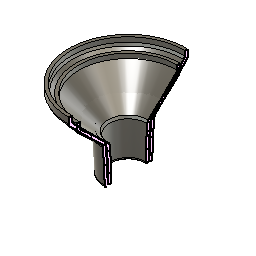
Násypky v4 (Autodesk Fusion 360 design; units mm, degrees)
Autodesk Fusion 360 part; units mm, degrees
sketch "Sketch1" plane through (0, 0, 0) normal (0, 0, 1) x (1, 0, 0)
  line L0 (16, 0) -> (17.25, 24)
  line L1 (17.25, 24) -> (40, 46.75)
  line L2 (17.25, 24) -> (32.4024, 24) construction
  line L3 (40, 46.75) -> (40, 51.75)
  line L4 (16, 0) -> (16, -1)
  line L5 (38, 47.5784) -> (38, 51.75)
  line L6 (15.2927, 24.8711) -> (38, 47.5784)
  line L7 (14, 0.052) -> (15.2927, 24.8711)
  line L8 (14, 0.052) -> (14, -1)
  line L9 (40, 51.75) -> (38, 51.75)
  line L10 (16, -1) -> (14, -1)
  dimension "d1" = 16
  dimension "d2" = 17.25
  dimension "d3" = 24
  dimension "d6" = 45
  dimension "d7" = 40
  dimension "d8" = 5
  dimension "d9" = 1
  dimension "d10" = -2
  constraint horizontal origin L0.start
  constraint horizontal L2
  constraint vertical L3
  constraint vertical L4
  measures "d1" horizontal distance of origin L0.start
  measures "d2" horizontal distance of origin L0.end
  measures "d3" vertical distance of origin L0.end
  measures "d6" angle of L1 L2
  measures "d7" horizontal distance of origin L1.end
  measures "d8" distance of L1.end L3.end
  measures "d9" distance of L0.start L4.end
revolve "Revolve1" add sketch "Sketch1" angle 360 about axis through (0, 1.75, 0) along (0, 1, 0) makes body 1
fillet "Fillet1" radius 4 1 edges at (-16.0826, 24, -6.2379) on bodies 1
fillet "Fillet2" radius 2 1 edges at (-37.2931, 46.75, -14.4646) on bodies 1
chamfer "Chamfer1" distance 1 angle 45 1 edges at (-14.2578, 24.8711, -5.5301) on bodies 1
chamfer "Chamfer2" distance 1 angle 45 1 edges at (-35.4284, 47.5784, -13.7414) on bodies 1
chamfer "Chamfer3" distance 0.3 angle 45 2 edges at (-13.0526, -1, -5.0626) (-14.9172, -1, -5.7858) on bodies 1
sketch "Sketch2" plane through (0, 0, 0) normal (0, 0, 1) x (1, 0, 0)
  line L0 (13.5, 0) -> (14.5, 22)
  line L1 (14.5, 22) -> (35, 40.7174)
  line L2 (35, 40.7174) -> (35, 45.7174)
  line L3 (13.5, 0) -> (13.5, -1)
  line L4 (33, 41.5995) -> (33, 45.7174)
  line L5 (12.5397, 22.9184) -> (33, 41.5995)
  line L6 (11.5, 0.0454) -> (12.5397, 22.9184)
  line L7 (11.5, 0.0454) -> (11.5, -1)
  line L8 (13.5, -1) -> (11.5, -1)
  line L9 (33, 45.7174) -> (35, 45.7174)
  dimension "d19" = 135
  dimension "d20" = 5
  dimension "d21" = 13.5
  dimension "d22" = 14.5
  dimension "d23" = 22
  dimension "d24" = 35
  dimension "d25" = 1
  dimension "d26" = -2
  constraint vertical L2
  constraint vertical L3
  constraint horizontal origin L0.start
  constraint perpendicular L2 L9
  measures "d19" angle of L0 L1
  measures "d20" distance of L1.end L2.end
  measures "d21" distance of origin L0.start
  measures "d22" horizontal distance of origin L0.end
  measures "d23" vertical distance of origin L0.end
  measures "d24" horizontal distance of origin L1.end
  measures "d25" distance of L0.start L3.end
revolve "Revolve2" add sketch "Sketch2" angle 360 about axis through (0, 1.75, 0) along (0, 1, 0) separate body makes body 2
chamfer "Chamfer4" distance 0.3 angle 45 2 edges at (-10.7218, -1, -4.1586) (-12.5864, -1, -4.8818) on bodies 2
fillet "Fillet3" radius 4 1 edges at (-13.5187, 22, -5.2434) on bodies 2
fillet "Fillet4" radius 2 1 edges at (-32.6315, 40.7174, -12.6565) on bodies 2
chamfer "Chamfer5" distance 1 angle 45 2 edges at (-30.7668, 41.5995, -11.9333) (-11.6911, 22.9184, -4.5345) on bodies 2
equation "d1 = ( 32 / 2 ) * 1 mm"
equation "d2 = ( 34.5 / 2 ) * 1 mm"
equation "d7 = ( 80 / 2 ) * 1 mm"
equation "d19 = 45 deg + 90 deg"
equation "d21 = ( 27 / 2 ) * 1 mm"
equation "d22 = ( 29 / 2 ) * 1 mm"
equation "d24 = ( 70 / 2 ) * 1 mm"
named bodies: "Násypka velká", "Násypka malá"
